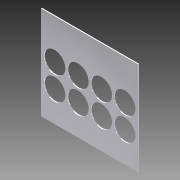
# Autodesk Inventor part: vessel support top
Saved by Autodesk Inventor 2011 (Build 150239000, 239)
## iProperties
Created: 2013-10-30
Part Number: vessel support top
Material: Default
Document SubType Name: Sheet Metal
Designer: Devon
Density: 1 g/cm^3
Sheet Metal Rule: Default
Author: Devon
Autodesk Inventor part; units mm, degrees
ref_plane "YZ Plane" through (0, 0, 0) normal (1, 0, 0) x (0, 1, 0)
ref_plane "XZ Plane" through (0, 0, 0) normal (0, 1, 0) x (-1, 0, 0)
ref_plane "XY Plane" through (0, 0, 0) normal (0, 0, 1) x (1, 0, 0)
sketch "Sketch1" plane through (0, 0, 0) normal (0, 0, 1) x (1, 0, 0)
  line L0 (-41.9595, 102.9157) -> (590.5005, 102.9157)
  line L1 (590.5005, 102.9157) -> (590.5005, 712.5157)
  line L2 (590.5005, 712.5157) -> (-41.9595, 712.5157)
  line L3 (-41.9595, 712.5157) -> (-41.9595, 102.9157)
  line L4 (-41.9595, 712.5157) -> (-23.3159, 712.5157)
  line L5 (590.5005, 712.5157) -> (546.0505, 712.5157)
  line L6 (546.0505, 712.5157) -> (406.3505, 712.5157)
  line L7 (406.3505, 712.5157) -> (393.6505, 712.5157)
  line L8 (393.6505, 712.5157) -> (253.9505, 712.5157)
  line L9 (253.9505, 712.5157) -> (241.2505, 712.5157)
  line L10 (241.2505, 712.5157) -> (101.5505, 712.5157)
  line L11 (101.5505, 712.5157) -> (88.8505, 712.5157)
  line L12 (88.8505, 712.5157) -> (-23.3159, 712.5157)
  line L13 (590.5005, 102.9157) -> (590.5005, 229.9157)
  line L14 (590.5005, 229.9157) -> (590.5005, 369.6157)
  line L15 (590.5005, 369.6157) -> (590.5005, 382.3157)
  line L16 (590.5005, 382.3157) -> (590.5005, 522.0157)
  circle A0 centre (46.5341, 452.1657) radius 69.85
  circle A1 centre (198.9341, 452.1657) radius 69.85
  circle A2 centre (351.3341, 452.1657) radius 69.85
  circle A3 centre (503.7341, 452.1657) radius 69.85
  circle A4 centre (46.5341, 299.7657) radius 69.85
  circle A5 centre (198.9341, 299.7657) radius 69.85
  circle A6 centre (351.3341, 299.7657) radius 69.85
  circle A7 centre (503.7341, 299.7657) radius 69.85
  line L17 (-23.3159, 712.5157) -> (116.3841, 712.5157)
  line L18 (116.3841, 712.5157) -> (129.0841, 712.5157)
  line L19 (129.0841, 712.5157) -> (268.7841, 712.5157)
  line L20 (268.7841, 712.5157) -> (281.4841, 712.5157)
  line L21 (281.4841, 712.5157) -> (421.1841, 712.5157)
  line L22 (421.1841, 712.5157) -> (433.8841, 712.5157)
  line L23 (433.8841, 712.5157) -> (573.5841, 712.5157)
  dimension "d0" = 632.46
  dimension "d1" = 609.6
  dimension "d2" = 18.6436
  dimension "d24" = 127
  dimension "d25" = 139.7
  dimension "d26" = 12.7
  dimension "d27" = 139.7
  dimension "d28" = 139.7
  dimension "d29" = 139.7
  dimension "d30" = 139.7
  dimension "d31" = 139.7
  dimension "d32" = 139.7
  dimension "d33" = 139.7
  dimension "d34" = 139.7
  dimension "d35" = 139.7
  dimension "d38" = 139.7
  dimension "d39" = 12.7
  dimension "d40" = 139.7
  dimension "d41" = 12.7
  dimension "d42" = 139.7
  dimension "d43" = 12.7
  dimension "d44" = 139.7
  constraints: 46 end point, 11 point on line, 8 centre point, 2 horizontal, 1 collinear, 1 parallel, 1 perpendicular, 11 other
  measures "d0" distance of L3.start L1.end
  measures "d1" distance of L1.end L0.end
  measures "d2" distance of L3.start L4.end
  measures "d24" distance of L0.end L13.end
  measures "d25" distance of L13.end L14.end
  measures "d26" distance of L14.end L15.end
  measures "d27" distance of L15.end L16.end
  measures "d28" diameter of A0
  measures "d29" diameter of A1
  measures "d30" diameter of A2
  measures "d31" diameter of A3
  measures "d32" diameter of A4
  measures "d33" diameter of A5
  measures "d34" diameter of A6
  measures "d35" diameter of A7
  measures "d38" distance of L4.end L17.end
  measures "d39" distance of L17.end L18.end
  measures "d40" distance of L18.end L19.end
  measures "d41" distance of L19.end L20.end
  measures "d42" distance of L20.end L21.end
  measures "d43" distance of L21.end L22.end
  measures "d44" distance of L22.end L23.end
extrude "Extrusion2" add sketch "Sketch1" along normal blind 6.35
equation "\"BendRadius\" = Thickness"
equation "\"BendReliefWidth\" = Thickness"
equation "\"BendReliefDepth\" = 0.5 * Thickness"
equation "\"CornerReliefSize\" = 4 * Thickness"
equation "\"MinimumRemnant\" = 2 * Thickness"
equation "\"TransitionRadius\" = BendRadius"
equation "\"JacobiRadiusSize\" = BendRadius"
equation "\"GapSize\" = Thickness"
equation "\"Thickness\" = 3.048"
body "Solid2"
